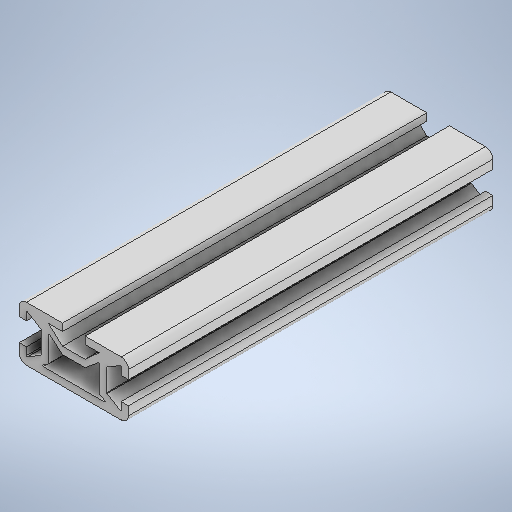
# Autodesk Inventor part: profile_15x60
Saved by Autodesk Inventor 2025.2 (Build 292293000, 293)
## iProperties
Created: 2025-04-03
Part Number: profile_15x60
Material: Generic
Document SubType Name: Modeling
Designer: kenne
Density: 1 g/cm^3
Appearance: Default
Author: kenne
Autodesk Inventor part; units mm, degrees
ref_plane "YZ Plane" through (0, 0, 0) normal (1, 0, 0) x (0, 1, 0)
ref_plane "XZ Plane" through (0, 0, 0) normal (0, 1, 0) x (-1, 0, 0)
ref_plane "XY Plane" through (0, 0, 0) normal (0, 0, 1) x (1, 0, 0)
sketch "Sketch1" plane through (0, 0, 0) normal (0, 0, 1) x (1, 0, 0)
  line L0 (-15, 7.5) -> (15, 7.5) construction
  line L1 (0, 11.0799) -> (0, -11.0799) projected
  line L2 (-15, 7.5) -> (-15, -7.5) construction
  line L3 (-15, 3.1) -> (-15, -3.1) construction
  line L4 (-15, 7.5) -> (-15, 3.1) construction
  line L5 (-15, 7.5) -> (-3.1, 7.5) construction
  line L6 (-15, 3.1) -> (-13, 3.1)
  line L7 (-3.1, 5.5) -> (-3.1, 7.5)
  line L8 (-13, 3.1) -> (-13, 5.5) construction
  line L9 (-15, 3.1) -> (-9, 3.1) construction
  line L10 (-13, 5.5) -> (-9, 3.1) construction
  line L11 (-9, 0) -> (-9, 3.1)
  line L12 (-21.4971, 0) -> (21.0828, 0) projected
  line L13 (-9, 0) -> (-9, -3.1) construction
  line L14 (-9, -3.1) -> (-13, -5.5) construction
  line L15 (-13, -5.5) -> (-13, -3.1) construction
  line L16 (-13, -3.1) -> (-15, -3.1)
  line L17 (-15, -3.1) -> (-15, -7.5) construction
  line L18 (-15, -7.5) -> (0, -7.5) construction
  line L19 (0, -7.5) -> (0, -5.5)
  line L20 (0, -5.5) -> (-9.1127, -5.5) construction
  line L21 (-9.1127, -5.5) -> (-7, -4.2324) construction
  line L22 (-7, -4.2324) -> (-7, 3.2725) construction
  line L23 (0, 0) -> (-3.1, 0)
  line L24 (-7, 3.2725) -> (-3.1, 0) construction
  line L25 (-3.1, 5.5) -> (-7, 5.5)
  line L26 (-7, 5.5) -> (-3.1, 1.9884)
  line L27 (-3.1, 1.9884) -> (0, 1.9884)
  line L28 (0, 1.9884) -> (0, 0)
  arc A0 (-13, 7.5) -> (-15, 5.5) centre (-13, 5.5) ccw
  line L29 (-13, 7.5) -> (-3.1, 7.5)
  line L30 (-15, 5.5) -> (-15, 3.1)
  arc A1 (-12.6971, 5.3183) -> (-13, 5.1468) centre (-12.8, 5.1468) ccw
  line L31 (-13, 5.1468) -> (-13, 3.1)
  line L32 (-12.6971, 5.3183) -> (-9, 3.1)
  arc A2 (-13, -5.1468) -> (-12.6971, -5.3183) centre (-12.8, -5.1468) ccw
  line L33 (-13, -5.1468) -> (-13, -3.1)
  line L34 (-12.6971, -5.3183) -> (-9, -3.1) construction
  arc A3 (-15, -5.5) -> (-13, -7.5) centre (-13, -5.5) ccw
  line L35 (-15, -5.5) -> (-15, -3.1)
  line L36 (-13, -7.5) -> (0, -7.5)
  arc A4 (-8.4935, -5.1285) -> (-8.3906, -5.5) centre (-8.3906, -5.3) ccw
  line L37 (-8.4935, -5.1285) -> (-7, -4.2324) construction
  line L38 (-8.3906, -5.5) -> (0, -5.5)
  arc A5 (-7.0971, -4.2906) -> (-7, -4.1191) centre (-7.2, -4.1191) ccw
  line L39 (-8.4935, -5.1285) -> (-7.0971, -4.2906)
  line L40 (-7, -4.1191) -> (-7, 3.2725) construction
  arc A6 (-9.0971, -3.1583) -> (-9, -2.9868) centre (-9.2, -2.9868) ccw
  line L41 (-9, -2.9868) -> (-9, 0)
  line L42 (-9.0971, -3.1583) -> (-12.6971, -5.3183)
  arc A7 (-6.6714, 2.9968) -> (-7, 2.8436) centre (-6.8, 2.8436) ccw
  line L43 (-7, -4.1191) -> (-7, 2.8436)
  line L44 (-3.1, 0) -> (-6.6714, 2.9968)
  line L45 (-3.1, 0) -> (0, 0)
  point P0 (0, 7.5)
  point P1 (-15, 0)
  dimension "d0" = 7.5
  dimension "d1" = 30
  dimension "d2" = 15
  dimension "d3" = 6.2
  dimension "d4" = 3.1
  dimension "d5" = 2
  dimension "d6" = 2.4
  dimension "d7" = 6
  dimension "d8" = 3.1
  dimension "d9" = 2
  dimension "d10" = 2
  dimension "d11" = 2
  dimension "d12" = 50
  dimension "d13" = 2
  dimension "outer_angle" = 2
  dimension "inner_angle" = 0.2
  dimension "d18" = 0.2
  dimension "d19" = 2
  dimension "d20" = 0.2
  dimension "d21" = 0.2
  dimension "d22" = 0.2
  dimension "d23" = 0.2
  constraints: 88 end point, 24 point on line, 17 tangent, 16 point on circle, 14 collinear, 8 centre point, 8 horizontal, 7 vertical, 4 vertical alignment, 3 equal length, 3 midpoint, 2 perpendicular, 1 parallel
  measures "d0" distance from line of L0 L23.start
  measures "d1" distance of L0.start L0.end
  measures "d2" distance of L0.start L2.end
  measures "d3" distance of L3.start L3.end
  measures "d4" distance from line of L1 L5.end
  measures "d5" distance of L3.start L6.end
  measures "d6" distance of L6.end L8.end
  measures "d7" distance of L3.start L9.end
  measures "d8" distance of L11.start L13.end
  measures "d9" distance of L18.end L19.end
  measures "d10" distance between parallel lines of L21 L14
  measures "d11" distance between parallel lines of L22 L11
  measures "d12" angle of L22 L24
  measures "d13" angle of L24 L26
  measures "outer_angle" radius of A0
  measures "inner_angle" radius of A1
  measures "d18" radius of A2
  measures "d19" radius of A3
  measures "d20" radius of A4
  measures "d21" radius of A5
  measures "d22" radius of A6
  measures "d23" radius of A7
extrude "Extrusion2" add sketch "Sketch1" along normal mid plane 100 contours L1 L12 L44 A7 L43 L11 L32 A1 L31 L6 L30 A0 L29 L7 L25 L26 L27 | L1 L36 A3 L35 L16 L33 A2 L42 A6 L41 L12 L43 A5 L39 A4 L38
mirror "Mirror2" about plane through (0, 0, 0) normal (1, 0, 0) of "Extrusion2"
equation "\"d18\" = inner_angle"
equation "\"d19\" = outer_angle"
equation "\"d20\" = inner_angle"
equation "\"d21\" = inner_angle"
equation "\"d22\" = inner_angle"
equation "\"d23\" = inner_angle"
body "Solid2"
